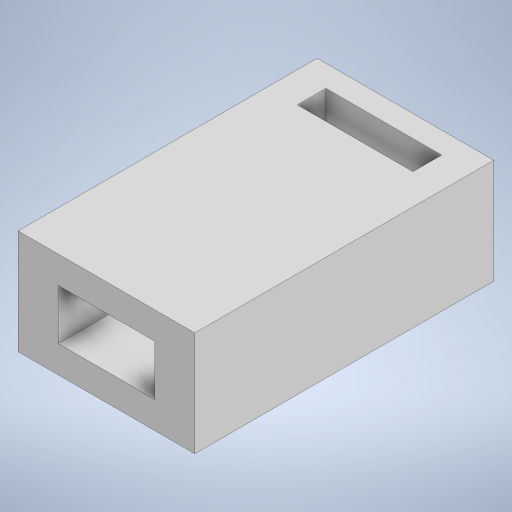
# Autodesk Inventor part: techo2
Saved by Autodesk Inventor 2023 (Build 270158000, 158)
## iProperties
Created: 2024-08-02
Part Number: techo2
Material: Generic
Document SubType Name: Modeling
Designer: sebas
Density: 1 g/cm^3
Appearance: Default
Author: sebas
Autodesk Inventor part; units mm, degrees
ref_plane "YZ Plane" through (0, 0, 0) normal (1, 0, 0) x (0, 1, 0)
ref_plane "XZ Plane" through (0, 0, 0) normal (0, 1, 0) x (-1, 0, 0)
ref_plane "XY Plane" through (0, 0, 0) normal (0, 0, 1) x (1, 0, 0)
sketch "Sketch1" plane through (0, 0, 0) normal (0, 1, 0) x (-1, 0, 0)
  line L0 (65, 0) -> (65, -110)
  line L1 (65, -110) -> (0, -110)
  line L2 (0, -110) -> (0, 0)
  line L3 (65, 0) -> (65, -34.9842)
  line L4 (65, 0) -> (50.25, 0)
  line L5 (50.25, 0) -> (50.25, -30.5)
  line L6 (0, 0) -> (14.75, 0)
  line L7 (14.75, 0) -> (14.75, -30.5)
  line L8 (50.25, -30.5) -> (14.75, -30.5)
  line L9 (0, 0) -> (14.75, 0)
  line L10 (50.25, 0) -> (65, 0)
  dimension "d0" = 65
  dimension "d1" = 110
  dimension "d2" = 14.75
  dimension "d3" = 30.5
  dimension "d4" = 14.75
  dimension "d5" = 30.5
  constraints: 22 end point, 4 horizontal, 2 perpendicular, 1 point on line, 1 vertical
  measures "d0" distance of L2.end L0.start
  measures "d1" distance of L0.start L0.end
  measures "d2" distance of L0.start L4.end
  measures "d3" distance of L4.end L5.end
  measures "d4" distance of L2.end L6.end
  measures "d5" distance of L6.end L7.end
extrude "Extrusion1" add sketch "Sketch1" along normal blind 18.5
sketch "Sketch2" plane through (0, 18.5, 0) normal (0, 1, 0) x (1, 0, 0)
  line L0 (0, 110) -> (-65, 110) projected
  line L1 (-65, 110) -> (-65, 0)
  line L2 (-14.75, 0) -> (0, 0) projected
  line L3 (-65, 0) -> (0, 0)
  line L4 (0, 0) -> (0, 110)
  line L5 (-65, 110) -> (-65, 0) projected
  line L6 (0, 110) -> (-65, 110)
  constraints: 8 end point, 3 perpendicular, 1 vertical
extrude "Extrusion2" add sketch "Sketch2" along normal blind 10
sketch "Sketch3" plane through (0, 0, 0) normal (0, -1, 0) x (1, 0, 0)
  line L0 (0, 0) -> (0, -110) projected
  line L1 (0, -110) -> (-65, -110) projected
  line L2 (0, 0) -> (0, -110)
  line L3 (0, -110) -> (-65, -110)
  line L4 (-65, -110) -> (-65, 0) projected
  line L5 (-65, -110) -> (-65, 0)
  line L6 (-65, 0) -> (0, 0)
  constraints: 8 end point, 3 perpendicular, 1 collinear
extrude "Extrusion3" add sketch "Sketch3" along normal blind 10
sketch "Sketch4" plane through (0, -10, 0) normal (0, -1, 0) x (1, 0, 0)
  line L0 (0, 0) -> (0, -110) projected
  line L1 (0, -110) -> (0, -102)
  line L2 (0, -110) -> (-32.5, -110)
  line L3 (-32.5, -110) -> (-24.5, -110)
  line L4 (0, -110) -> (-65, -110) projected
  line L5 (-32.5, -110) -> (-32.5, -102)
  line L6 (-32.5, -102) -> (-11.25, -102)
  line L7 (-11.25, -102) -> (-11.25, -91.5)
  line L8 (-11.25, -91.5) -> (-53.75, -91.5)
  line L9 (-53.75, -91.5) -> (-53.75, -102)
  line L10 (-53.75, -102) -> (-32.5, -102)
  dimension "d19" = 32.5
  dimension "d26" = 8
  dimension "d27" = 21.25
  dimension "d28" = 10.5
  dimension "d29" = 42.5
  dimension "d30" = 10.5
  constraints: 18 end point, 3 perpendicular, 3 point on line, 1 collinear, 1 vertical
  measures "d19" distance of L0.end L2.end
  measures "d26" distance of L2.end L5.end
  measures "d27" distance of L5.end L6.end
  measures "d28" distance of L6.end L7.end
  measures "d29" distance of L7.end L8.end
  measures "d30" distance of L8.end L9.end
extrude "Extrusion4" cut sketch "Sketch4" against normal through all
body "Solid1"
